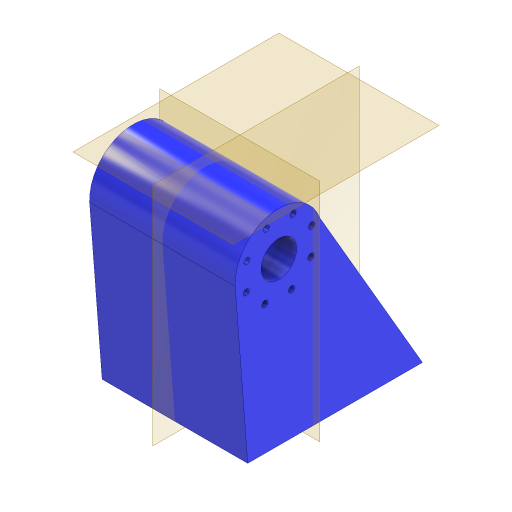
# Autodesk Inventor part: Ушко петли крышки
Saved by Autodesk Inventor 2023.2 (Build 272271030, 271C)
## iProperties
Created: 2025-04-30
Part Number: Ушко петли крышки
Material: Типовые
Document SubType Name: Modeling
Designer: Олег Коноваленко
Density: 1 g/cm^3
Appearance: Синий — малярная краска — глянцевая
Author: Олег Коноваленко
Autodesk Inventor part; units mm, degrees
sketch "Эскиз1" plane through (0, 0, 0) normal (1, 0, 0) x (0, 1, 0)
  line L0 (-84.2261, 0) -> (14.4739, 0) construction
  circle A0 centre (-14.6261, 11.6003) radius 15 projected
  line L1 (-70.1261, -37.7219) -> (-70.1261, 22.2781)
  line L2 (-70.1261, -37.7219) -> (-9.6116, -2.5367)
  line L3 (-15.295, 26.5854) -> (-70.1261, 22.2781)
  line L4 (-70.1261, 36.1012) -> (-70.1261, -83.8988) projected
  line L5 (-70.1261, -37.7219) -> (-60.535, -54.2175)
  line L6 (-15.295, 26.5854) -> (-16.485, 41.7343)
  circle A1 centre (-10.3011, 0.4068) radius 1.05 projected
  circle A2 centre (-19.4828, 0.6271) radius 1.05 projected
  circle A3 centre (-25.8196, 7.2753) radius 1.05 projected
  circle A4 centre (-25.5993, 16.4571) radius 1.05 projected
  circle A5 centre (-18.9511, 22.7938) radius 1.05 projected
  circle A6 centre (-9.7693, 22.5736) radius 1.05 projected
  circle A7 centre (-3.4326, 15.9253) radius 1.05 projected
  circle A8 centre (-3.6528, 6.7436) radius 1.05 projected
  circle A9 centre (-14.6261, 11.6003) radius 6.1
  dimension "d21" = 60
  dimension "d24" = 70
  dimension "d25" = 55
  dimension "d26" = 59.825
  dimension "d29" = 12.2
  constraints: 10 end point, 2 perpendicular, 2 point on circle, 1 centre point, 1 point on line, 1 vertical
  measures "d21" distance of L1.start L1.end
  measures "d24" distance from line of L2.end L5
  measures "d25" distance from line of L6 L1.end
  measures "d26" angle of L2 L1
  measures "d29" diameter of A9
extrude "Выдавливание3" add sketch "Эскиз1" along normal mid plane 50 contours A0 L3 | L2 L1 L3 A0 picked at (-14.2037, 20.8402)
sketch "Эскиз3" plane through (-25, -70.1261, -37.7219) normal (0, -1, 0) x (1, 0, 0)
  point P0 (25, 37.7219)
